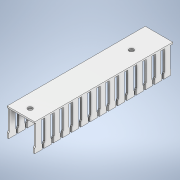
# Autodesk Inventor part: Cablecanal Ranurado 30 x 30 L=150
Saved by Autodesk Inventor 2020 (Build 240168000, 168)
## iProperties
Created: 2020-09-30
Part Number: Cablecanal Ranurado 30 x 30 L=150
Material: PVC-Piping
Document SubType Name: Modeling
Designer: Hernan
Density: 1.4 g/cm^3
Appearance: Smooth - White
Author: Hernan
Autodesk Inventor part; units mm, degrees
ref_plane "YZ Plane" through (0, 0, 0) normal (1, 0, 0) x (0, 1, 0)
ref_plane "XZ Plane" through (0, 0, 0) normal (0, 1, 0) x (-1, 0, 0)
ref_plane "XY Plane" through (0, 0, 0) normal (0, 0, 1) x (1, 0, 0)
sketch "Sketch1" plane through (0, 0, 0) normal (0, 0, 1) x (1, 0, 0)
  line L0 (-31.9903, -7.2804) -> (-1.9903, -7.2804)
  line L1 (-1.9903, -7.2804) -> (-1.9903, 22.7196)
  line L2 (-1.9903, 22.7196) -> (-31.9903, 22.7196)
  line L3 (-31.9903, -7.2804) -> (-31.9903, 22.7196)
  line L4 (-30.2903, 22.7196) -> (-30.2903, -7.2804)
  line L5 (-31.9903, -5.5804) -> (-1.9903, -5.5804)
  line L6 (-3.6903, 22.7196) -> (-3.6903, -7.2804)
  line L7 (-31.9903, 21.0196) -> (-1.9903, 21.0196)
  point P0 (0, 0)
  point P1 (0, 0)
  point P2 (-3.6903, 21.0196)
  point P3 (-30.2903, 21.0196)
  point P4 (-30.2903, -5.5804)
  point P5 (-3.6903, -5.5804)
  dimension "d0" = 30
  dimension "d1" = 30
  dimension "d2" = 1.7
  dimension "d3" = 1.7
  dimension "d4" = 1.7
  dimension "d5" = 1.7
  constraints: 16 end point, 8 point on line, 3 horizontal, 2 perpendicular, 2 vertical, 1 parallel
  measures "d0" distance of L0.start L0.end
  measures "d1" distance of L0.end L1.end
  measures "d2" distance between parallel lines of L0 L5
  measures "d3" distance between parallel lines of L3 L4
  measures "d4" distance between parallel lines of L1 L6
  measures "d5" distance between parallel lines of L2 L7
extrude "Extrusion1" add sketch "Sketch1" against normal blind 150
extrude "Extrusion2" cut sketch "Sketch1" against normal blind 150 contours L4 L5 L6 L0 | L4 L7 L6 L5
sketch "Boceto2" plane through (-31.9903, 22.7196, 0) normal (0, 1, 0) x (1, 0, 0)
  line L0 (28.3, 150) -> (1.7, 150) projected
  line L1 (0, 0) -> (30, 0) projected
  circle A0 centre (15, 120) radius 2.5
  circle A1 centre (15, 10) radius 2.5
  line L2 (30, 0) -> (30, 150) projected
  point P0 (31.9903, 0)
  dimension "d12" = 5
  dimension "d13" = 5
  dimension "d14" = 110
  dimension "d15" = 10
  dimension "d16" = 15
  dimension "d17" = 15
  constraints: 2 centre point
  measures "d12" diameter of A0
  measures "d13" diameter of A1
  measures "d14" distance of A1.centre A0.centre
  measures "d15" distance from line of L1 A1.centre
  measures "d16" distance from line of L2 A0.centre
  measures "d17" distance from line of L2 A1.centre
extrude "Extrusión3" cut sketch "Boceto2" against normal blind 10
sketch "Boceto3" plane through (-31.9903, -7.2804, 0) normal (-1, 0, 0) x (0, 0, 1)
  line L0 (0, 0) -> (-8, 0)
  line L1 (0, 0) -> (-150, 0) projected
  line L2 (-8, 0) -> (-8, 5)
  line L3 (0, 0) -> (0, 5)
  line L4 (0, 30) -> (0, 0) projected
  line L5 (-1, 6.5) -> (-1, 28.3)
  line L6 (0, 30) -> (-150, 30) projected
  line L7 (-7, 6.5) -> (-7, 28.3)
  line L8 (-8, 5) -> (-7, 6.5)
  line L9 (-1, 6.5) -> (0, 5)
  line L10 (-10, 0) -> (-18, 0)
  line L11 (-18, 0) -> (-18, 5)
  line L12 (-10, 0) -> (-10, 5)
  line L13 (-11, 6.5) -> (-11, 28.3)
  line L14 (-17, 6.5) -> (-17, 28.3)
  line L15 (-18, 5) -> (-17, 6.5)
  line L16 (-11, 6.5) -> (-10, 5)
  line L17 (-20, 0) -> (-28, 0)
  line L18 (-28, 0) -> (-28, 5)
  line L19 (-20, 0) -> (-20, 5)
  line L20 (-21, 6.5) -> (-21, 28.3)
  line L21 (-27, 6.5) -> (-27, 28.3)
  line L22 (-28, 5) -> (-27, 6.5)
  line L23 (-21, 6.5) -> (-20, 5)
  line L24 (-30, 0) -> (-38, 0)
  line L25 (-38, 0) -> (-38, 5)
  line L26 (-30, 0) -> (-30, 5)
  line L27 (-31, 6.5) -> (-31, 28.3)
  line L28 (-37, 6.5) -> (-37, 28.3)
  line L29 (-38, 5) -> (-37, 6.5)
  line L30 (-31, 6.5) -> (-30, 5)
  line L31 (-40, 0) -> (-48, 0)
  line L32 (-48, 0) -> (-48, 5)
  line L33 (-40, 0) -> (-40, 5)
  line L34 (-41, 6.5) -> (-41, 28.3)
  line L35 (-47, 6.5) -> (-47, 28.3)
  line L36 (-48, 5) -> (-47, 6.5)
  line L37 (-41, 6.5) -> (-40, 5)
  line L38 (-50, 0) -> (-58, 0)
  line L39 (-58, 0) -> (-58, 5)
  line L40 (-50, 0) -> (-50, 5)
  line L41 (-51, 6.5) -> (-51, 28.3)
  line L42 (-57, 6.5) -> (-57, 28.3)
  line L43 (-58, 5) -> (-57, 6.5)
  line L44 (-51, 6.5) -> (-50, 5)
  line L45 (-60, 0) -> (-68, 0)
  line L46 (-68, 0) -> (-68, 5)
  line L47 (-60, 0) -> (-60, 5)
  line L48 (-61, 6.5) -> (-61, 28.3)
  line L49 (-67, 6.5) -> (-67, 28.3)
  line L50 (-68, 5) -> (-67, 6.5)
  line L51 (-61, 6.5) -> (-60, 5)
  line L52 (-70, 0) -> (-78, 0)
  line L53 (-78, 0) -> (-78, 5)
  line L54 (-70, 0) -> (-70, 5)
  line L55 (-71, 6.5) -> (-71, 28.3)
  line L56 (-77, 6.5) -> (-77, 28.3)
  line L57 (-78, 5) -> (-77, 6.5)
  line L58 (-71, 6.5) -> (-70, 5)
  line L59 (-80, 0) -> (-88, 0)
  line L60 (-88, 0) -> (-88, 5)
  line L61 (-80, 0) -> (-80, 5)
  line L62 (-81, 6.5) -> (-81, 28.3)
  line L63 (-87, 6.5) -> (-87, 28.3)
  line L64 (-88, 5) -> (-87, 6.5)
  line L65 (-81, 6.5) -> (-80, 5)
  line L66 (-90, 0) -> (-98, 0)
  line L67 (-98, 0) -> (-98, 5)
  line L68 (-90, 0) -> (-90, 5)
  line L69 (-91, 6.5) -> (-91, 28.3)
  line L70 (-97, 6.5) -> (-97, 28.3)
  line L71 (-98, 5) -> (-97, 6.5)
  line L72 (-91, 6.5) -> (-90, 5)
  line L73 (-100, 0) -> (-108, 0)
  line L74 (-108, 0) -> (-108, 5)
  line L75 (-100, 0) -> (-100, 5)
  line L76 (-101, 6.5) -> (-101, 28.3)
  line L77 (-107, 6.5) -> (-107, 28.3)
  line L78 (-108, 5) -> (-107, 6.5)
  line L79 (-101, 6.5) -> (-100, 5)
  line L80 (-110, 0) -> (-118, 0)
  line L81 (-118, 0) -> (-118, 5)
  line L82 (-110, 0) -> (-110, 5)
  line L83 (-111, 6.5) -> (-111, 28.3)
  line L84 (-117, 6.5) -> (-117, 28.3)
  line L85 (-118, 5) -> (-117, 6.5)
  line L86 (-111, 6.5) -> (-110, 5)
  line L87 (-120, 0) -> (-128, 0)
  line L88 (-128, 0) -> (-128, 5)
  line L89 (-120, 0) -> (-120, 5)
  line L90 (-121, 6.5) -> (-121, 28.3)
  line L91 (-121, 6.5) -> (-120, 5)
  line L92 (-127.0613, 6.5) -> (-127.0613, 28.3)
  line L93 (0, 28.3) -> (-150, 28.3) projected
  line L94 (0, 28.3) -> (-150, 28.3)
  line L95 (-150, 0) -> (-150, 28.3)
  line L96 (-150, 30) -> (-150, 0) projected
  line L97 (0, 28.3) -> (0, 5)
  line L98 (0, 0) -> (0, 30) projected
  line L99 (-128, 0) -> (-150, 0)
  line L100 (-128, 0) -> (-128, 5)
  line L101 (-128, 5) -> (-127.0613, 6.5)
  line L102 (-138, 0) -> (-138, 5)
  line L103 (-131, 6.5) -> (-131, 28.3)
  line L104 (-131, 6.5) -> (-130, 5)
  line L105 (-130, 0) -> (-130, 5)
  line L106 (-130, 0) -> (-138, 0)
  line L107 (-137.0613, 6.5) -> (-137.0613, 28.3)
  line L108 (-138, 0) -> (-138, 5)
  line L109 (-138, 5) -> (-137.0613, 6.5)
  line L110 (-148, 0) -> (-148, 5)
  line L111 (-141, 6.5) -> (-141, 28.3)
  line L112 (-141, 6.5) -> (-140, 5)
  line L113 (-140, 0) -> (-140, 5)
  line L114 (-140, 0) -> (-148, 0)
  line L115 (-147.0613, 6.5) -> (-147.0613, 28.3)
  line L116 (-148, 0) -> (-148, 5)
  line L117 (-148, 5) -> (-147.0613, 6.5)
  point P0 (0, 7.2804)
  point P1 (-10, 0)
  point P2 (-20, 0)
  point P3 (-18, 0)
  point P4 (-30, 0)
  point P5 (-28, 0)
  point P6 (-38, 0)
  point P7 (-48, 0)
  point P8 (-58, 0)
  point P9 (-68, 0)
  point P10 (-78, 0)
  point P11 (-88, 0)
  point P12 (-98, 0)
  point P13 (-110, 0)
  point P14 (-108, 0)
  point P15 (-120, 0)
  point P16 (-118, 0)
  point P17 (-128, 0)
  point P18 (-141, 28.3)
  point P19 (-147.0613, 28.3)
  point P20 (-148, 0)
  point P21 (-140, 0)
  point P22 (-131, 28.3)
  point P23 (-137.0613, 28.3)
  point P24 (-138, 0)
  point P25 (-130, 0)
  dimension "d20" = 8
  dimension "d26" = 8
  dimension "d27" = 8
  dimension "d29" = 8
  dimension "d30" = 8
  dimension "d31" = 8
  dimension "d32" = 8
  dimension "d33" = 8
  dimension "d34" = 8
  dimension "d35" = 8
  dimension "d36" = 8
  dimension "d37" = 8
  dimension "d38" = 8
  dimension "d40" = 2
  dimension "d41" = 2
  dimension "d42" = 2
  dimension "d43" = 2
  dimension "d44" = 2
  dimension "d45" = 2
  dimension "d46" = 2
  dimension "d47" = 2
  dimension "d48" = 2
  dimension "d49" = 2
  dimension "d50" = 4
  dimension "d51" = 4
  dimension "d54" = 8
  dimension "d55" = 8
  dimension "d56" = 2
  dimension "d57" = 2
  constraints: 222 end point, 5 collinear, 1 horizontal, 1 perpendicular, 1 point on line, 1 vertical, 32 other
  measures "d20" distance of L0.start L0.end
  measures "d26" distance of L12.start L11.start
  measures "d27" distance of L19.start L18.start
  measures "d29" distance of L26.start L25.start
  measures "d30" distance of L33.start L32.start
  measures "d31" distance of L40.start L39.start
  measures "d32" distance of L47.start L46.start
  measures "d33" distance of L54.start L53.start
  measures "d34" distance of L61.start L60.start
  measures "d35" distance of L68.start L67.start
  measures "d36" distance of L75.start L74.start
  measures "d37" distance of L82.start L81.start
  measures "d38" distance of L89.start L88.start
  measures "d40" distance of L12.start L0.end
  measures "d41" distance of L19.start L11.start
  measures "d42" distance of L26.start L18.start
  measures "d43" distance between parallel lines of L33 L25
  measures "d44" distance between parallel lines of L40 L32
  measures "d45" distance between parallel lines of L47 L39
  measures "d46" distance between parallel lines of L54 L46
  measures "d47" distance between parallel lines of L61 L53
  measures "d48" distance between parallel lines of L68 L60
  measures "d49" distance between parallel lines of L67 L75
  measures "d50" distance between parallel lines of L83 L77
  measures "d51" distance between parallel lines of L90 L84
  measures "d54" distance of L106.start L106.end
  measures "d55" distance of L114.start L114.end
  measures "d56" distance of L106.start L88.start
  measures "d57" distance of L114.start L106.end
extrude "Extrusión4" cut sketch "Boceto3" against normal blind 30 contours L1 L12 L16 L13 L93 L7 L8 L2 | L9 L5 L93 L4 | L1 L19 L23 L20 L93 L14 L15 L11 | L1 L26 L30 L27 L93 L21 L22 L18 | L93 L115 L117 L110 L1 L95 | L93 L111 L112 L113 L1 L110 L117 L115 | L1 L33 L37 L34 L93 L28 L29 L25 | L93 L107 L109 L102 L1 L113 L112 L111 | L93 L103 L104 L105 L1 L102 L109 L107 | L1 L40 L44 L41 L93 L35 L36 L32 | L93 L92 L101 L88 L1 L105 L104 L103 | L1 L47 L51 L48 L93 L42 L43 L39 | L93 L84 L85 L81 L1 L89 L91 L90 | L1 L54 L58 L55 L93 L49 L50 L46 | L93 L77 L78 L74 L1 L82 L86 L83 | L1 L61 L65 L62 L93 L56 L57 L53 | L93 L70 L71 L67 L1 L75 L79 L76 | L1 L68 L72 L69 L93 L63 L64 L60
extrude "Extrusión5" add sketch "Boceto3" against normal blind 30 contours L93 L111 L112 L113 L1 L110 L117 L115 | L93 L103 L104 L105 L1 L102 L109 L107
sketch "Boceto4" plane through (-31.9903, -7.2804, -148) normal (0, -1, 0) x (1, 0, 0)
  line L0 (1.7, 20) -> (1.7, 28) projected
  line L1 (1.7, 20) -> (1.7, -3.5053)
  line L2 (28.3, 20) -> (28.3, -3.5053)
  line L3 (28.3, -3.5053) -> (1.7, -3.5053)
  line L4 (1.7, 20) -> (28.3, 20)
  line L5 (0, 18) -> (30, 18) projected
  point P0 (31.9903, 148)
  constraints: 8 end point, 2 vertical, 1 parallel, 1 perpendicular
extrude "Extrusión6" cut sketch "Boceto4" against normal blind 28.3
body "Solid1"
